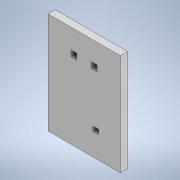
# Autodesk Inventor part: ds input capture cover v1
Saved by Autodesk Inventor 2020 (Build 240168000, 168)
## iProperties
Created: 2020-06-17
Part Number: ds input capture cover v1
Material: Generic
Document SubType Name: Modeling
Designer: Arjun Oberoi
Density: 1 g/cm^3
Appearance: Default
Author: Arjun Oberoi
Autodesk Inventor part; units mm, degrees
ref_plane "YZ Plane" through (0, 0, 0) normal (1, 0, 0) x (0, 1, 0)
ref_plane "XZ Plane" through (0, 0, 0) normal (0, 1, 0) x (-1, 0, 0)
ref_plane "XY Plane" through (0, 0, 0) normal (0, 0, 1) x (1, 0, 0)
sketch "Sketch1" plane through (0, 0, 0) normal (0, 0, 1) x (1, 0, 0)
  line L0 (0, 0) -> (17, 0)
  line L1 (17, 0) -> (17, 31)
  line L2 (17, 31) -> (0, 31)
  line L3 (0, 31) -> (0, 0)
  dimension "d0" = 17
  dimension "d1" = 31
  constraints: 8 end point, 2 parallel, 1 horizontal, 1 perpendicular
  measures "d0" distance of L2.end L1.end
  measures "d1" distance of L1.end L0.end
extrude "Extrusion1" add sketch "Sketch1" along normal blind 1.5
sketch "Sketch2" plane through (0, 0, 1.5) normal (0, 0, 1) x (1, 0, 0)
  line L0 (17, 31) -> (0, 31) projected
  line L1 (2.5, 31) -> (14.5, 31)
  line L2 (14.5, 31) -> (14.5, 5)
  line L3 (14.5, 5) -> (2.5, 5)
  line L4 (2.5, 5) -> (2.5, 31)
  line L5 (0, 0) -> (17, 0) projected
  line L6 (4.5, 0) -> (12.5, 0)
  line L7 (12.5, 0) -> (12.5, 5)
  line L8 (12.5, 5) -> (4.5, 5)
  line L9 (4.5, 5) -> (4.5, 0)
  line L10 (0, 31) -> (0, 0) projected
  point P0 (4.5, 5)
  dimension "d4" = 12
  dimension "d5" = 8
  dimension "d6" = 5
  dimension "d7" = 17
  dimension "d8" = 2.5
  dimension "d9" = 4.5
  constraints: 16 end point, 4 parallel, 2 horizontal, 2 perpendicular, 2 point on line, 1 collinear
  measures "d4" distance of L2.end L3.end
  measures "d5" distance of L8.end L7.end
  measures "d6" distance of L7.end L6.end
  measures "d7" distance of L0.start L0.end
  measures "d8" distance between parallel lines of L10 L4
  measures "d9" distance between parallel lines of L10 L9
extrude "Extrusion2" cut sketch "Sketch2" against normal up to surface (1.5 mm away) contours L2 L3 L4 L0 | L7 L5 L9 L3
sketch "Sketch3" plane through (0, 0, 1.5) normal (0, 0, 1) x (1, 0, 0)
  line L0 (-4, 35) -> (21, 35)
  line L1 (21, 35) -> (21, 0)
  line L2 (21, 0) -> (-4, 0)
  line L3 (-4, 0) -> (-4, 35)
  line L4 (2.5, 31) -> (0, 31) projected
  line L5 (0, 31) -> (0, 0) projected
  line L6 (17, 0) -> (17, 31) projected
  line L7 (0, 0) -> (4.5, 0) projected
  dimension "d12" = 4
  dimension "d13" = 4
  dimension "d14" = 4
  constraints: 8 end point, 2 parallel, 1 collinear, 1 horizontal, 1 perpendicular
  measures "d12" distance between parallel lines of L0 L4
  measures "d13" distance between parallel lines of L3 L5
  measures "d14" distance between parallel lines of L6 L1
extrude "Extrusion3" add sketch "Sketch3" along normal blind 2.5
sketch "Sketch4" plane through (0, 0, 1.5) normal (0, 0, -1) x (-1, 0, 0)
  line L0 (0, 0) -> (-4.5, 0) projected
  line L1 (-4.5, 0) -> (-12.5, 0)
  line L2 (-12.5, 0) -> (-12.5, 5)
  line L3 (-12.5, 5) -> (-4.5, 5)
  line L4 (-4.5, 5) -> (-4.5, 0)
  constraints: 8 end point, 2 parallel, 1 horizontal, 1 perpendicular
extrude "Extrusion4" cut sketch "Sketch4" against normal blind 1
sketch "Sketch5" plane through (0, 0, 1.5) normal (0, 0, -1) x (-1, 0, 0)
  line L0 (-11.5, 7.75) -> (-13.5, 7.75)
  line L1 (-13.5, 7.75) -> (-13.5, 9.25)
  line L2 (-13.5, 9.25) -> (-11.5, 9.25)
  line L3 (-11.5, 9.25) -> (-11.5, 7.75)
  line L4 (-12.5, 5) -> (-4.5, 5) projected
  line L5 (-4.5, 5) -> (-4.5, 0) projected
  line L6 (-12.5, 0) -> (-12.5, 5) projected
  point P0 (0, 0)
  dimension "d19" = 2
  dimension "d20" = 1.5
  dimension "d21" = 2.75
  dimension "d25" = 1
  constraints: 8 end point, 2 parallel, 1 horizontal, 1 perpendicular
  measures "d19" distance of L1.end L2.end
  measures "d20" distance of L0.end L1.end
  measures "d21" distance between parallel lines of L0 L4
  measures "d25" distance between parallel lines of L6 L3
extrude "Extrusion5" cut sketch "Sketch5" against normal through all
sketch "Sketch6" plane through (0, 0, 1.5) normal (0, 0, -1) x (-1, 0, 0)
  line L0 (-4, 26.25) -> (-6, 26.25)
  line L1 (-6, 26.25) -> (-6, 28.25)
  line L2 (-6, 28.25) -> (-4, 28.25)
  line L3 (-4, 28.25) -> (-4, 26.25)
  line L4 (-2.5, 31) -> (0, 31) projected
  line L5 (-2.5, 5) -> (-2.5, 31) projected
  line L6 (0, 31) -> (0, 0) projected
  line L7 (-12.5, 5) -> (-4.5, 5) projected
  line L8 (-8.5, 5) -> (-8.5, 35)
  line L9 (-21, 35) -> (4, 35) projected
  line L10 (-13, 26.25) -> (-11, 26.25)
  line L11 (-11, 26.25) -> (-11, 28.25)
  line L12 (-11, 28.25) -> (-13, 28.25)
  line L13 (-13, 28.25) -> (-13, 26.25)
  dimension "d26" = 2.75
  dimension "d27" = 2
  dimension "d28" = 2
  dimension "d30" = 4
  constraints: 18 end point, 4 symmetric about line, 2 midpoint, 2 parallel, 1 horizontal, 1 perpendicular
  measures "d26" distance between parallel lines of L4 L2
  measures "d27" distance of L0.end L1.end
  measures "d28" distance between parallel lines of L1 L3
  measures "d30" distance between parallel lines of L6 L3
extrude "Extrusion6" cut sketch "Sketch6" against normal through all
equation "\"d8\" = -0.5 * d4 + 0.5 * d7"
equation "\"d9\" = -0.5 * d5 + 0.5 * d7"
body "Solid1"
